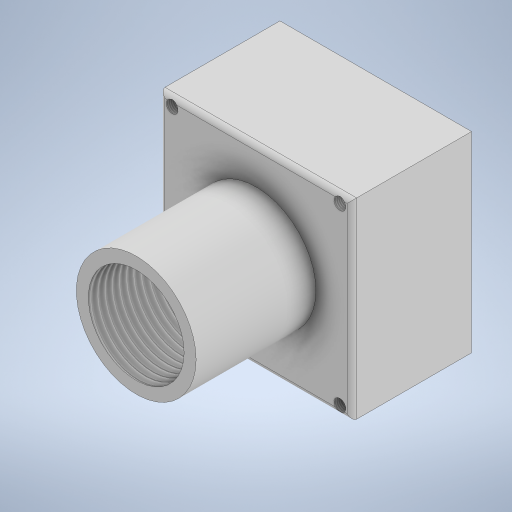
# Autodesk Inventor part: Lab 1
Saved by Autodesk Inventor 2024 (Build 280153000, 153)
## iProperties
Created: 2024-01-23
Part Number: Lab 1
Material: Genérico
Document SubType Name: Modeling
Designer: pazjo
Density: 1 g/cm^3
Appearance: Valor por defecto
Author: pazjo
Autodesk Inventor part; units mm, degrees
ref_plane "YZ Plane" through (0, 0, 0) normal (1, 0, 0) x (0, 1, 0)
ref_plane "XZ Plane" through (0, 0, 0) normal (0, 1, 0) x (-1, 0, 0)
ref_plane "XY Plane" through (0, 0, 0) normal (0, 0, 1) x (1, 0, 0)
sketch "Boceto1" plane through (0, 0, 0) normal (0, 0, 1) x (1, 0, 0)
  line L0 (-40, 40) -> (40, 40)
  line L1 (40, 40) -> (40, -40)
  line L2 (40, -40) -> (-40, -40)
  line L3 (-40, -40) -> (-40, 40)
  line L4 (-40, 40) -> (40, -40) construction
  line L5 (40, 40) -> (-40, -40) construction
  point P0 (0, 0)
  dimension "d0" = 80
  dimension "d1" = 80
  constraints: 12 end point, 2 midpoint, 2 parallel, 1 horizontal, 1 perpendicular
  measures "d0" distance of L1.end L2.end
  measures "d1" distance of L0.end L1.end
extrude "Extrusión1" add sketch "Boceto1" along normal blind 50
sketch "Boceto2" plane through (0, 0, 50) normal (0, 0, 1) x (1, 0, 0)
  circle A0 centre (0, 0) radius 25
  circle A1 centre (0, 0) radius 20
  dimension "d4" = 50
  dimension "d5" = 5
  constraints: 2 centre point, 1 coincident
  measures "d4" diameter of A0
  measures "d5" radial gap between concentric circles of A0 A1
extrude "Extrusión2" add sketch "Boceto2" along normal blind 50
sketch "Boceto3" plane through (0, 0, 0) normal (0, 0, -1) x (-1, 0, 0)
  line L0 (-40, 40) -> (40, 40) projected
  line L1 (40, 40) -> (40, -40) projected
  line L2 (-40, 40) -> (40, 40)
  line L3 (40, 40) -> (40, -40)
  line L4 (40, -40) -> (-40, -40)
  line L5 (-40, -40) -> (-40, 40)
  line L6 (-35, -36.4247) -> (35, 36.4247) construction
  line L7 (35, -36.4247) -> (-35, 36.4247) construction
  line L8 (-35, 36.4247) -> (-37.5, 36.4247)
  line L9 (-40, 36.4247) -> (-40, 40)
  line L10 (-40, 40) -> (-35, 40)
  line L11 (-35, 40) -> (-35, 38.9247)
  arc A0 (-35.0145, 36.4247) -> (-35.0108, 36.4359) centre (-35.2551, 36.5094) ccw
  circle A1 centre (-35, 36.4247) radius 2.5
  circle A2 centre (35, 36.4247) radius 2.5
  circle A3 centre (-35, -36.4247) radius 2.5
  circle A4 centre (35, -36.4247) radius 2.5
  line L12 (35, 36.4247) -> (32.5, 36.4247)
  line L13 (-32.5, 36.4247) -> (-35, 36.4247)
  line L14 (35, -36.4247) -> (35, -33.9247)
  line L15 (35, 33.9247) -> (35, 36.4247)
  line L16 (-35, 36.4247) -> (-35, 33.9247)
  line L17 (-35, -33.9247) -> (-35, -36.4247)
  line L18 (-35, -36.4247) -> (-32.5, -36.4247)
  line L19 (32.5, -36.4247) -> (35, -36.4247)
  point P0 (0, 0)
  point P1 (-38.2122, 38.2122)
  dimension "d9" = 70
  constraints: 36 end point, 12 parallel, 12 point on circle, 6 perpendicular, 5 centre point, 4 horizontal, 2 midpoint, 2 point on line, 1 tangent
  measures "d9" distance of L7.end L6.end
sketch "Boceto4" plane through (0, 0, 0) normal (0, 0, -1) x (-1, 0, 0)
  point P0 (0, 0)
extrude "Extrusión3" cut sketch "Boceto3" against normal blind 50 contours A1 L13 L8 | A1 L16 L13 | L8 L16 A1 | A2 L15 L12 | L12 L15 A2 | L18 L17 A3 | A3 L17 L18 | A4 L19 L14 | L14 L19 A4
thread "Rosca1" size "M5x0.8" class "6H" standard "ANSI Metric M Profile" full length
thread "Rosca2" size "M5x0.8" class "6H" standard "ANSI Metric M Profile" full length
thread "Rosca3" size "M5x0.8" class "6H" standard "ANSI Metric M Profile" full length
thread "Rosca4" size "M5x0.8" class "6H" standard "ANSI Metric M Profile" full length
fillet "Empalme1" radius 2 4 edges at (0, -40, 50) (40, 0, 50) (0, 40, 50) (-40, 0, 50)
thread "Rosca5" size "M40x3" class "6H" standard "ANSI Metric M Profile" full length
sketch "Boceto5" plane through (0, 0, 50) normal (0, 0, 1) x (1, 0, 0)
  circle A0 centre (0, 0) radius 20
  constraints: 1 centre point, 1 coincident
extrude "Extrusión4" add sketch "Boceto5" along normal blind 20
